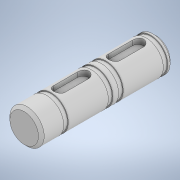
# Autodesk Inventor part: Shaft_stage_output
Saved by Autodesk Inventor 2020 (Build 240168000, 168)
## iProperties
Created: 2020-05-12
Part Number: Shaft_stage_output
Material: Generic
Document SubType Name: Sheet Metal
Designer: avi41
Density: 1 g/cm^3
Appearance: Default
Sheet Metal Rule: Default
Author: avi41
Autodesk Inventor part; units mm, degrees
ref_plane "YZ Plane" through (0, 0, 0) normal (1, 0, 0) x (0, 1, 0)
ref_plane "XY Plane" through (0, 0, 0) normal (0, 0, 1) x (1, 0, 0)
sketch "Sketch1" plane through (0, 0, 0) normal (0, 1, 0) x (-1, 0, 0)
  line L0 (0, -16.1) -> (0, 16.1) construction
  line L1 (-3.6, 0) -> (0.6, 0) construction
  line L2 (0, 11.5) -> (-3, 11.5)
  line L3 (-3, 11.5) -> (-3, -11.5)
  line L4 (-3, -11.5) -> (0, -11.5)
  line L5 (0, 11.5) -> (0, -11.5)
  point P0 (0, 0)
  dimension "d0" = 3
  dimension "d1" = 23
  constraints: 8 end point, 3 perpendicular, 2 point on line, 1 horizontal, 1 other
  measures "d0" distance of L3.end L4.end
  measures "d1" distance of L2.end L3.end
revolve "Revolution1" add sketch "Sketch1" angle 360 about axis through (0, 0, 11.5) along (0, 0, -1)
sketch "Sketch2" plane through (0, 0, 0) normal (0, 1, 0) x (-1, 0, 0)
  line L0 (3, -9.625) -> (-3, -9.625) construction
  line L1 (0, -16.1) -> (0, 16.1) construction
  line L2 (-4.2, 0) -> (4.2, 0) construction
  line L3 (-3, 6.8) -> (-2.85, 6.8)
  line L4 (-2.85, 6.8) -> (-2.85, 7.6)
  line L5 (-2.85, 7.6) -> (-3, 7.6)
  line L6 (-3, 7.6) -> (-3, 6.8)
  line L7 (3, -11.5) -> (-3, -11.5) projected
  line L8 (-3, 6.8) -> (-3, 7.6)
  line L9 (-3, -0.2) -> (-2.85, -0.2)
  line L10 (-2.85, -0.2) -> (-2.85, -1)
  line L11 (-2.85, -1) -> (-3, -1)
  line L12 (-3, -1) -> (-3, -0.2)
  line L13 (-3, -2) -> (-2.85, -2)
  line L14 (-2.85, -2) -> (-2.85, -2.8)
  line L15 (-2.85, -2.8) -> (-3, -2.8)
  line L16 (-3, -2.8) -> (-3, -2)
  line L17 (-3, -9.8) -> (-2.85, -9.8)
  line L18 (-2.85, -9.8) -> (-2.85, -10.6)
  line L19 (-2.85, -10.6) -> (-3, -10.6)
  line L20 (-3, -10.6) -> (-3, -9.8)
  line L21 (3, -11.5) -> (-3, -11.5) projected
  line L22 (3, 11.5) -> (-3, 11.5) projected
  line L23 (-3, -11.5) -> (-3, 11.5) projected
  dimension "d34" = 0.8
  dimension "d35" = 2.85
  dimension "d57" = 7
  dimension "d58" = 7
  dimension "d59" = 1
  dimension "d70" = 0.975
  constraints: 34 end point, 10 collinear, 8 parallel, 4 horizontal, 4 perpendicular, 1 other
  measures "d34" distance of L3.end L4.end
  measures "d35" distance between parallel lines of L1 L4
  measures "d57" distance between parallel lines of L3 L9
  measures "d58" distance from line of L17 L14.end
  measures "d59" distance between parallel lines of L11 L13
revolve "Revolution2" cut sketch "Sketch2" angle 360 about axis through (0, 0, 0) along (0, 0, 1)
ref_plane "Work Plane2" through (0, 3, 0) normal (0, 1, 0) x (-1, 0, 0)
sketch "Sketch4" plane through (0, 3, 0) normal (0, 1, 0) x (-1, 0, 0)
  line L0 (0, -16.1) -> (0, 16.1) construction
  line L1 (1, -8.375) -> (1, -4.225)
  line L2 (-1, -4.225) -> (-1, -8.375)
  arc A0 (-1, -8.375) -> (1, -8.375) centre (0, -8.375) ccw
  arc A1 (1, -4.225) -> (-1, -4.225) centre (0, -4.225) ccw
  line L3 (3, -11.5) -> (-3, -11.5) projected
  line L4 (-1, -6.3) -> (1, -6.3) construction
  line L5 (-3, -2.8) -> (3, -2.8) construction
  line L6 (3, -9.8) -> (-3, -9.8) construction
  line L7 (-3, -1) -> (3, -1) construction
  line L8 (3, -2) -> (-3, -2) construction
  line L9 (-3, -2) -> (-3, -1) projected
  line L10 (-3, -1.5) -> (3, -1.5) construction
  line L11 (1, 5.375) -> (1, 1.225)
  line L12 (-1, 1.225) -> (-1, 5.375)
  arc A2 (1, 5.375) -> (-1, 5.375) centre (0, 5.375) ccw
  arc A3 (-1, 1.225) -> (1, 1.225) centre (0, 1.225) ccw
  line L13 (-1, 3.3) -> (1, 3.3) construction
  point P0 (0, 0)
  dimension "d49" = 6.15
  dimension "d50" = 1
  dimension "d60" = 3.5
  dimension "d61" = 3.5
  constraints: 14 end point, 8 point on circle, 8 symmetric about line, 4 centre point, 3 midpoint, 3 tangent, 2 point on line, 1 horizontal, 1 parallel, 3 other
  measures "d50" radius of A0
  measures "d60" distance between parallel lines of L4 L6
  measures "d61" distance between parallel lines of L5 L4
extrude "Extrusion2" cut sketch "Sketch4" against normal blind 1
chamfer "Chamfer3" distance 0.5 angle 45 2 edges at (-3, 0, -11.5) (-3, 0, 11.5)
equation "\"module\" = 1"
equation "\"pressure_ang\" = 30deg"
equation "\"pitch\" = 3.1416 * module"
equation "\"addendum\" = 0.45 * module"
equation "\"dedendum\" = 0.65 * module"
equation "\"tooth_depth\" = addendum + dedendum"
equation "\"addendum_mod_shaft\" = 0.45 * module"
equation "\"root_fillet_r\" = 0.16 * module"
equation "\"addendum_mod_hub\" = -addendum_mod_shaft"
equation "\"nom_space_t_hub\" = nom_tooth_t_shaft"
equation "\"nom_tooth_t_shaft\" = 2.090415"
body "Solid1"
